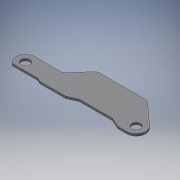
# Autodesk Inventor part: rinnku
Saved by Autodesk Inventor 2018 (Build 220112000, 112)
## iProperties
Created: 2016-08-23
Part Number: rinnku
Material: GFRP
Document SubType Name: Modeling
Designer: hiro
Density: 1.75 g/cm^3
Appearance: 滑らか - 淡い灰色
Mass: 9.22094 g
Surface Area: 59.6576 cm^2
Volume: 5.26911 cm^3
Author: hiro
Autodesk Inventor part; units mm, degrees
ref_plane "YZ Plane" through (0, 0, 0) normal (1, 0, 0) x (0, 1, 0)
ref_plane "XZ Plane" through (0, 0, 0) normal (0, 1, 0) x (-1, 0, 0)
ref_plane "XY Plane" through (0, 0, 0) normal (0, 0, 1) x (1, 0, 0)
sketch "スケッチ1" plane through (0, 0, 0) normal (0, 0, 1) x (1, 0, 0)
  line L0 (-50, 0) -> (50, 0) construction
  circle A0 centre (-50, 0) radius 4.05
  circle A1 centre (50, 0) radius 4.05
  line L1 (-50, 8.5) -> (50, 8.5)
  line L2 (-50, -8.5) -> (50, -8.5)
  arc A2 (-50, 8.5) -> (-50, -8.5) centre (-50, 0) ccw
  arc A3 (50, -8.5) -> (50, 8.5) centre (50, 0) ccw
  line L3 (55.697, 6.3082) -> (35, 25)
  line L4 (35, 25) -> (-10, 25)
  line L5 (-10, 25) -> (-24.9014, 8.5)
  line L6 (-16.3218, 18) -> (42.751, 18) construction
  line L7 (-10, 25) -> (-10, 18) construction
  line L8 (35, 25) -> (35, 18) construction
  circle A4 centre (32.5, 21.5) radius 1.55
  circle A5 centre (-7.5, 21.5) radius 1.55
  circle A6 centre (12.5, 21.5) radius 1.55
  line L9 (-10, 21.5) -> (35, 21.5) construction
  line L10 (35, 24) -> (-10, 24) construction
  line L11 (-10, 24) -> (-10, 19) construction
  line L12 (-10, 19) -> (35, 19) construction
  line L13 (35, 19) -> (35, 24) construction
  point P0 (0, 0)
  point P1 (0, 0)
  dimension "d0" = 100
  dimension "d1" = 8.1
  dimension "d2" = 8.5
  dimension "d8" = 8.1
  dimension "d10" = 7
  dimension "d11" = 45
  dimension "d12" = 2.5
  dimension "d13" = 3.1
  dimension "d14" = 2.5
  dimension "d15" = 15
  dimension "d17" = 5
  dimension "d18" = 19
  constraints: 28 end point, 9 point on line, 7 centre point, 6 horizontal, 5 coincident, 5 midpoint, 5 point on circle, 4 perpendicular, 4 tangent, 2 equal radius, 2 parallel
  measures "d0" distance of L0.start L0.end
  measures "d1" diameter of A0
  measures "d2" radius of A2
  measures "d8" diameter of A1
  measures "d10" distance between parallel lines of L4 L6
  measures "d11" distance between parallel lines of L8 L7
  measures "d12" distance from line of A5.centre L7
  measures "d13" diameter of A5
  measures "d14" distance from line of L8 A4.centre
  measures "d15" distance from line of L8 L0.end
  measures "d17" distance between parallel lines of L10 L12
  measures "d18" distance between parallel lines of L0 L12
extrude "押し出し1" add sketch "スケッチ1" along normal blind 2
fillet "フィレット1" radius 5 3 edges at (-24.9014, 8.5, 1) (-10, 25, 1) (35, 25, 1)
sketch "スケッチ2" plane through (0, 0, 2) normal (0, 0, 1) x (1, 0, 0)
  arc A0 (50, -8.5) -> (55.697, 6.3082) centre (50, 0) ccw projected
  line L0 (18, -20) -> (-35.4549, -20) construction
  line L1 (-76.9607, -11.5) -> (-72, -11.5)
  line L2 (-72, -11.5) -> (-62, -7)
  line L3 (-62, -7) -> (-32, -7)
  line L4 (-32, -7) -> (-22, -11.5)
  line L5 (-22, -11.5) -> (-17.0393, -11.5)
  line L6 (-17.0393, -11.5) -> (-17.0393, -12.4)
  line L7 (-17.0393, -12.4) -> (-76.9607, -12.4)
  line L8 (-76.9607, -12.4) -> (-76.9607, -11.5)
  line L9 (-31.9893, -6.95) -> (-62.0107, -6.95)
  line L10 (-62.0107, -6.95) -> (-72.0107, -11.45)
  line L11 (-72.0107, -11.45) -> (-77.0107, -11.45)
  line L12 (-77.0107, -11.45) -> (-77.0107, -12.45)
  line L13 (-77.0107, -12.45) -> (-16.9893, -12.45)
  line L14 (-16.9893, -12.45) -> (-16.9893, -11.45)
  line L15 (-16.9893, -11.45) -> (-21.9893, -11.45)
  line L16 (-21.9893, -11.45) -> (-31.9893, -6.95)
  circle A1 centre (-50, 0) radius 4.05 projected
  circle A2 centre (-50, 0) radius 5.5 construction
  circle A3 centre (50, 0) radius 4.05 projected
  line L17 (83.3205, -17.7128) -> (50, 0) construction
  line L18 (50, 0) -> (18, -20) construction
  line L19 (83.3205, -17.7128) -> (37.8533, -17.7128) construction
  line L20 (-11.6402, -10.1128) -> (48.2812, -10.1128)
  line L21 (48.2812, -10.1128) -> (48.2812, -9.2128)
  line L22 (48.2812, -9.2128) -> (43.3205, -9.2128)
  line L23 (43.3205, -9.2128) -> (33.3205, -4.7128)
  line L24 (33.3205, -4.7128) -> (3.3205, -4.7128)
  line L25 (3.3205, -4.7128) -> (-6.6795, -9.2128)
  line L26 (-6.6795, -9.2128) -> (-11.6402, -9.2128)
  line L27 (-11.6402, -9.2128) -> (-11.6402, -10.1128)
  line L28 (-6.6902, -9.1628) -> (3.3098, -4.6628)
  line L29 (3.3098, -4.6628) -> (33.3312, -4.6628)
  line L30 (33.3312, -4.6628) -> (43.3312, -9.1628)
  line L31 (43.3312, -9.1628) -> (48.3312, -9.1628)
  line L32 (48.3312, -9.1628) -> (48.3312, -10.1628)
  line L33 (48.3312, -10.1628) -> (-11.6902, -10.1628)
  line L34 (-11.6902, -10.1628) -> (-11.6902, -9.1628)
  line L35 (-11.6902, -9.1628) -> (-6.6902, -9.1628)
  point P0 (0, 0)
  dimension "d19" = 20
  dimension "d20" = 32
  dimension "d21" = 40
  dimension "d22" = 10
  dimension "d23" = 8.5
  dimension "d24" = 10
  dimension "d25" = 30
  dimension "d26" = 13
  dimension "d27" = 0.05
  dimension "d32" = 11
  dimension "d33" = 120
  dimension "d34" = 1
  dimension "d36" = 5
  dimension "d37" = 40
  dimension "d38" = 8.5
  dimension "d39" = 0.05
  constraints: 72 end point, 10 perpendicular, 9 equal length, 6 horizontal, 4 collinear, 2 horizontal alignment, 2 parallel, 1 centre point, 1 coincident, 14 other
  measures "d19" vertical distance of A0.centre L0.start
  measures "d20" horizontal distance of L0.start A0.centre
  measures "d21" horizontal distance of L0.start L4.end
  measures "d22" horizontal distance of L4.end L3.end
  measures "d23" distance from line of L0.start L5
  measures "d24" horizontal distance of L1.end L2.end
  measures "d25" distance of L2.end L3.end
  measures "d26" distance from line of L0.start L3
  measures "d27" distance between parallel lines of L9 L3
  measures "d32" diameter of A2
  measures "d33" angle of L18 L17
  measures "d34" distance of L13.end L14.end
  measures "d36" distance from line of L14 L15.end
  measures "d37" horizontal distance of L17.start L22.end
  measures "d38" distance from line of L22 L17.start
  measures "d39" distance between parallel lines of L28 L25
extrude "押し出し2" cut sketch "スケッチ2" against normal blind 10 contours L1 L2 L3 L4 L5 L6 L7 L8 | L16 L15 L14 L13 L12 L11 L10 L9 | L27 L26 L25 L24 L23 L22 L21 L20 | L28 L29 L30 L31 L32 L33 L34 L35
fillet "フィレット2" radius 2 7 edges at (-28.5448, -8.5, 1) (-31.9893, -6.95, 1) (-5.2173, -8.5, 1) (3.3098, -4.6628, 1) (41.8583, -8.5, 1) (33.3312, -4.6628, 1) (-54.8936, -6.95, 1)
sketch "スケッチ3" plane through (0, 0, 0) normal (0, 0, -1) x (-1, 0, 0)
  circle A0 centre (7.5, 21.5) radius 1.55 projected
  circle A1 centre (7.5, 21.5) radius 1.55
  circle A2 centre (-12.5, 21.5) radius 1.55 projected
  circle A3 centre (-12.5, 21.5) radius 1.55
  circle A4 centre (-32.5, 21.5) radius 1.55 projected
  circle A5 centre (-32.5, 21.5) radius 1.55
  point P0 (0, 0)
  constraints: 3 centre point, 3 coincident
extrude "押し出し3" add sketch "スケッチ3" against normal up to surface (2 mm away)
equation "\"d8\" = d1"
equation "\"d14\" = d12"
equation "\"d24\" = d22"
equation "\"d37\" = d21"
equation "\"d38\" = d23"
